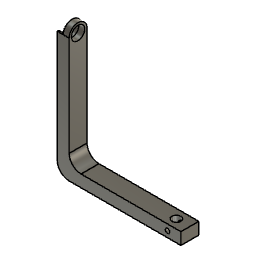
Pos23 (Autodesk Fusion 360 design; units mm, degrees)
Autodesk Fusion 360 part; units mm, degrees
sketch "Sketch1" plane through (0, 0, 0) normal (0, 1, 0) x (1, 0, 0)
  line L0 (8, 0) -> (83, 0)
  line L1 (83, 0) -> (83, -8)
  line L2 (83, -8) -> (16, -8)
  line L3 (8, -16) -> (8, -89)
  line L4 (8, -89) -> (4, -89)
  line L5 (4, -89) -> (4, -83)
  line L6 (4, -83) -> (0, -83)
  line L7 (0, -83) -> (0, -8)
  arc A0 (16, -8) -> (8, -16) centre (16, -16) ccw
  arc A1 (8, 0) -> (0, -8) centre (8, -8) ccw
  line L8 (74, 0) -> (74, -4) construction
  circle A2 centre (74, -4) radius 1.5
  dimension "d1" = 83
  dimension "d2" = 8
  dimension "d3" = 4
  dimension "d4" = 8
  dimension "d5" = 8
  dimension "d6" = 8
  dimension "d7" = 89
  dimension "d8" = 83
  dimension "d9" = 75
  dimension "d11" = 4
  dimension "d12" = 3
  dimension "d13" = 66
  constraint horizontal L0
  constraint perpendicular L0 L1
  constraint perpendicular L1 L2
  constraint perpendicular L2 L3
  constraint perpendicular L3 L4
  constraint perpendicular L4 L5
  constraint perpendicular L5 L6
  constraint perpendicular L0 L7
  constraint tangent L2 A0
  constraint tangent L3 A0
  constraint coincident origin L0
  constraint tangent L0 A1
  constraint tangent L7 A1
  constraint coincident L0 L8.start
  constraint perpendicular L0 L8
  constraint coincident L8.end A2.centre
  measures "d1" distance of origin L0.end
  measures "d2" distance of L0.end L1.end
  measures "d3" distance of L3.end L4.end
  measures "d4" distance of L3 L7
  measures "d5" radius of A0
  measures "d6" radius of A1
  measures "d7" distance of L0 L4
  measures "d8" distance of L0 L6
  measures "d9" distance of L1 L3
  measures "d11" distance of L8.start L8.end
  measures "d12" diameter of A2
  measures "d13" distance of L3 L8.end
extrude "Extrude1" add sketch "Sketch1" along normal blind 12
fillet "Fillet1" radius 6 1 edges at (6, 0, 89)
fillet "Fillet2" radius 6 1 edges at (6, 12, 89)
sketch "Sketch2" plane through (0, 0, 0) normal (1, 0, 0) x (0, 1, 0)
  arc A0 (12, 83) -> (0, 83) centre (6, 83) ccw
  line L0 (0, 83) -> (0, 16)
  line L1 (0, 16) -> (12, 16)
  line L2 (12, 16) -> (12, 83)
  line L3 (6, 16) -> (6, 83) construction
  circle A1 centre (6, 83) radius 4.5
  line L4 (0, 8) -> (0, 83)
  line L5 (0, 83) -> (12, 83)
  line L6 (12, 83) -> (12, 8)
  line L7 (12, 8) -> (0, 8)
  dimension "d20" = 67
  dimension "d21" = 9
  constraint midpoint L1 L3.start
  constraint perpendicular L1 L3
  constraint coincident A0.centre L3.end
  measures "d20" distance of L3.start A0.centre
  measures "d21" diameter of A1
hole "Hole1" at (0, 6, 83) direction (1, 0, 0) diameter 9 depth 13 tip angle 118 counterbore diameter 10 counterbore depth 4
sketch "Sketch3" plane through (0, 0, 8) normal (0, 0, 1) x (-1, 0, 0)
  line L0 (-16, 0) -> (-83, 0)
  line L1 (-83, 0) -> (-83, -12)
  line L2 (-83, -12) -> (-16, -12)
  line L3 (-16, -12) -> (-16, 0)
  line L4 (-83, -6) -> (-74, -6) construction
  circle A0 centre (-74, -6) radius 3
  dimension "d27" = 9
  dimension "d28" = 6
  constraint midpoint L1 L4.start
  constraint perpendicular L1 L4
  constraint coincident L4.end A0.centre
  measures "d27" distance of L4.start L4.end
  measures "d28" diameter of A0
hole "Hole2" at (74, 6, 8) direction (0, 0, -1) diameter 6 depth 13 tip angle 118
